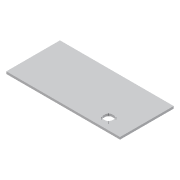
# Autodesk Inventor part: Lid_TopPanel
Saved by Autodesk Inventor 2016 (Build 200138000, 138)
## iProperties
Created: 2014-10-15
Part Number: Lid_TopPanel
Material: Polycarbonat, klar
Document SubType Name: Modeling
Designer: Gero Hofmann
Density: 1.2 g/cm^3
Appearance: Polycarbonat - klar
Author: Gero Hofmann
Autodesk Inventor part; units mm, degrees
ref_plane "YZ Plane" through (0, 0, 0) normal (1, 0, 0) x (0, 1, 0)
ref_plane "XZ Plane" through (0, 0, 0) normal (0, 1, 0) x (-1, 0, 0)
ref_plane "XY Plane" through (0, 0, 0) normal (0, 0, 1) x (1, 0, 0)
sketch "Skizze1" plane through (0, 0, 0) normal (0, 0, 1) x (1, 0, 0)
  line L0 (-250, 120) -> (250, 120)
  line L1 (250, 120) -> (250, -120)
  line L2 (250, -120) -> (-250, -120)
  line L3 (-250, -120) -> (-250, 120)
  line L4 (-250, 120) -> (250, -120) construction
  line L5 (250, 120) -> (-250, -120) construction
  point P0 (0, 0)
  dimension "d0" = 500
  dimension "d1" = 240
  constraints: 12 end point, 2 midpoint, 2 parallel, 1 horizontal, 1 perpendicular
  measures "d0" distance of L1.end L2.end
  measures "d1" distance of L0.end L1.end
extrude "Extrusion1" add sketch "Skizze1" along normal blind 10
sketch "Skizze3" plane through (0, 0, 0) normal (0, 0, -1) x (-1, 0, 0)
  line L0 (-250, 120) -> (-250, -120) projected
  line L1 (-250, -120) -> (250, -120) projected
  line L2 (-156.245, -89) -> (-143.755, -89)
  line L3 (-131, -76.245) -> (-131, -63.755)
  line L4 (-143.755, -51) -> (-156.245, -51)
  line L5 (-169, -63.755) -> (-169, -76.245)
  line L6 (-156.245, -89) -> (-143.755, -51) construction
  line L7 (-131, -76.245) -> (-169, -63.755) construction
  arc A0 (-143.755, -89) -> (-131, -76.245) centre (-150, -70) ccw
  arc A1 (-169, -76.245) -> (-156.245, -89) centre (-150, -70) ccw
  arc A2 (-131, -63.755) -> (-143.755, -51) centre (-150, -70) ccw
  arc A3 (-156.245, -51) -> (-169, -63.755) centre (-150, -70) ccw
  point P0 (0, 0)
  dimension "d32" = 38
  dimension "d33" = 20
  dimension "d34" = 50
  dimension "d35" = 100
  constraints: 12 end point, 8 point on circle, 4 centre point, 3 concentric, 2 midpoint, 2 parallel, 2 perpendicular, 1 horizontal
  measures "d32" distance between parallel lines of L2 L4
  measures "d33" radius of A2
  measures "d34" distance from line of L1 A3.centre
  measures "d35" distance from line of L0 A3.centre
extrude "Extrusion3" cut sketch "Skizze3" against normal through all
sketch "Skizze4" plane through (0, 0, 0) normal (0, 0, -1) x (-1, 0, 0)
  arc A0 (-143.755, -89) -> (-131, -76.245) centre (-150, -70) ccw projected
  line L0 (-134, -86) -> (-166, -86)
  line L1 (-166, -86) -> (-166, -54)
  line L2 (-166, -54) -> (-134, -54)
  line L3 (-134, -54) -> (-134, -86)
  line L4 (-134, -86) -> (-166, -54) construction
  line L5 (-166, -86) -> (-134, -54) construction
  point P0 (0, 0)
  dimension "d38" = 32
  dimension "d39" = 32
  constraints: 12 end point, 2 midpoint, 2 parallel, 1 horizontal, 1 perpendicular
  measures "d38" distance of L1.end L2.end
  measures "d39" distance of L0.end L1.end
hole "Bohrung3" at (134, -54, 0) at (134, -86, 0) at (166, -86, 0) at (166, -54, 0) direction (0, 0, 1) diameter 2.459 end through all thread size "M3x0.5" class "6H" standard "ISO Metric profile"
